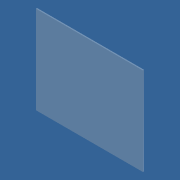
# Autodesk Inventor part: top plate
Saved by Autodesk Inventor 2012 (Build 160160000, 160)
## iProperties
Created: 2012-03-16
Part Number: top plate
Material: Polycarbonate, Clear
Document SubType Name: Modeling
Designer: Ed
Mass: 1937.93 g
Surface Area: 5215.15 cm^2
Volume: 1614.95 cm^3
Density: 1.2 g/cm^3
Author: Ed
Autodesk Inventor part; units mm, degrees
ref_plane "YZ Plane" through (0, 0, 0) normal (1, 0, 0) x (0, 1, 0)
ref_plane "XZ Plane" through (0, 0, 0) normal (0, 1, 0) x (-1, 0, 0)
ref_plane "XY Plane" through (0, 0, 0) normal (0, 0, 1) x (1, 0, 0)
sketch "Sketch1" plane through (0, 0, 0) normal (0, 0, 1) x (1, 0, 0)
  line L0 (0, 0) -> (556.26, 0)
  line L1 (556.26, 0) -> (556.26, 457.2)
  line L2 (556.26, 457.2) -> (0, 457.2)
  line L3 (0, 457.2) -> (0, 0)
  dimension "d0" = 457.2
  dimension "d1" = 556.26
  constraints: 8 end point, 2 parallel, 1 horizontal, 1 perpendicular
  measures "d0" distance of L2.end L0.start
  measures "d1" distance of L0.start L0.end
extrude "Extrusion1" add sketch "Sketch1" along normal blind 6.35
body "Solid1"
